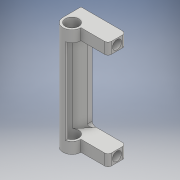
# Autodesk Inventor part: MousetrapFront
Saved by Autodesk Inventor 2018.3 (Build 223284000, 284)
## iProperties
Created: 2018-07-01
Part Number: MousetrapFront
Material: Generic
Document SubType Name: Modeling
Designer: mzhang
Density: 1 g/cm^3
Appearance: Default
Author: mzhang
Autodesk Inventor part; units mm, degrees
ref_plane "YZ Plane" through (0, 0, 0) normal (1, 0, 0) x (0, 1, 0)
ref_plane "XZ Plane" through (0, 0, 0) normal (0, 1, 0) x (-1, 0, 0)
ref_plane "XY Plane" through (0, 0, 0) normal (0, 0, 1) x (1, 0, 0)
sketch "Sketch1" plane through (0, 0, 0) normal (0, 0, 1) x (1, 0, 0)
  circle A0 centre (0, 0) radius 6
  arc A1 (-8, 0) -> (8, 0) centre (0, 0) ccw
  line L0 (-8, 8) -> (-8, 0)
  line L1 (32, 16) -> (8, 16)
  line L2 (8, 0) -> (32, 0)
  line L3 (32, 0) -> (32, 16)
  line L4 (8, 16) -> (-8, 16)
  line L5 (-8, 16) -> (-8, 8)
  point P0 (20, 8)
  dimension "d0" = 12
  dimension "d1" = 2
  constraints: 12 end point, 2 centre point, 2 horizontal, 2 point on circle, 1 coincident, 1 parallel, 1 perpendicular
  measures "d0" diameter of A0
  measures "d1" radial gap between concentric circles of A0 A1
extrude "Extrusion1" add sketch "Sketch1" along normal blind 95.9
sketch "Sketch2" plane through (-8, 16, 0) normal (0, 1, 0) x (1, 0, 0)
  line L0 (40, 0) -> (0, 0) projected
  line L1 (0, 0) -> (0, -95.9) projected
  line L2 (40, -95.9) -> (0, -95.9) projected
  line L3 (40, 0) -> (40, -95.9) projected
  line L4 (10, -85.9) -> (10, -10)
  line L5 (10, -10) -> (30, -10)
  line L6 (30, -85.9) -> (10, -85.9)
  line L7 (30, -85.9) -> (40, -85.9)
  line L8 (30, -10) -> (40, -10)
  line L9 (40, 0) -> (40, -95.9) projected
  point P0 (8, 0)
  dimension "d5" = 10
  constraints: 10 end point, 2 perpendicular, 2 point on line, 1 other
  measures "d5" distance between parallel lines of L2 L6
extrude "Extrusion2" cut sketch "Sketch2" against normal blind 95.9 contours L3 L7 L6 L4 L5 L8
sketch "Sketch3" plane through (32, 0, 0) normal (1, 0, 0) x (0, 0, -1)
  line L0 (-10, 16) -> (-10, 0) projected
  line L1 (0, 0) -> (-10, 0) projected
  line L2 (0, 0) -> (0, 16) projected
  line L3 (0, 16) -> (-10, 16) projected
  line L4 (-85.9, 0) -> (-85.9, 16) projected
  line L5 (-85.9, 16) -> (-95.9, 16) projected
  line L6 (-95.9, 0) -> (-95.9, 16) projected
  line L7 (-85.9, 0) -> (-95.9, 0) projected
  circle A0 centre (-90.9, 8) radius 4
  circle A1 centre (-5, 8) radius 4
  dimension "d9" = 8
  dimension "d10" = 8
  constraints: 2 centre point
  measures "d9" diameter of A0
  measures "d10" diameter of A1
extrude "Extrusion3" cut sketch "Sketch3" against normal blind 15 contours A0 | A1
chamfer "Chamfer1" distance 6 angle 45 1 edges at (2, 5.6569, 47.95)
fillet "Fillet1" radius 3 2 edges at (2, 13.8284, 10) (2, 13.8284, 85.9)
fillet "Fillet2" radius 3 4 edges at (32, 0, 90.9) (32, 16, 90.9) (32, 16, 5) (32, 0, 5)
body "Solid1"
